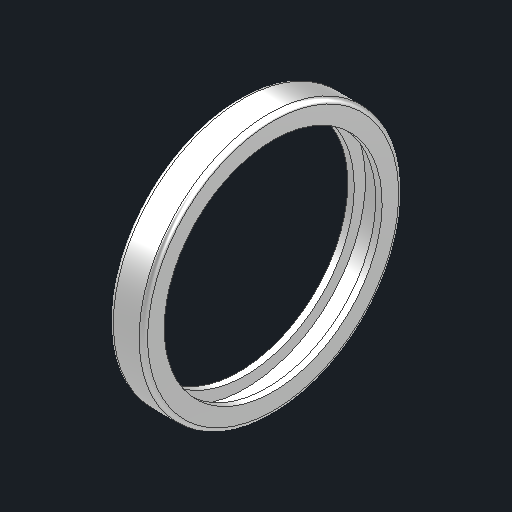
# Autodesk Inventor part: Rubber Wheel Cap
Saved by Autodesk Inventor 2026.2 (Build 302298000, 298)
## iProperties
Created: 2024-10-29
Part Number: Rubber Wheel Cap
Material: Generic
Document SubType Name: Modeling
Designer: Ethan
Density: 1 g/cm^3
Appearance: Default
Author: Ethan
Autodesk Inventor part; units mm, degrees
ref_plane "YZ Plane" through (0, 0, 0) normal (1, 0, 0) x (0, 1, 0)
ref_plane "XZ Plane" through (0, 0, 0) normal (0, 1, 0) x (-1, 0, 0)
ref_plane "XY Plane" through (0, 0, 0) normal (0, 0, 1) x (1, 0, 0)
sketch "Sketch1" plane through (0, 0, 0) normal (1, 0, 0) x (0, 1, 0)
  circle A0 centre (0, 0) radius 30.25
  circle A1 centre (0, 0) radius 25.4
  dimension "d0" = 60.5
  dimension "d3" = 50.8
  constraints: 2 centre point, 2 coincident
  measures "d0" diameter of A0
  measures "d3" diameter of A1
extrude "Extrusion1" add sketch "Sketch1" along normal mid plane 8
sketch "Sketch2" plane through (0, 0, 0) normal (1, 0, 0) x (0, 1, 0)
  circle A0 centre (0, 0) radius 28
  dimension "d4" = 56
  constraints: 1 centre point, 1 coincident
  measures "d4" diameter of A0
extrude "Extrusion2" cut sketch "Sketch2" along normal mid plane 5
fillet "Fillet1" radius 1 2 edges at (-4, -30.25, 0) (4, -30.25, 0)
body "Solid1"
